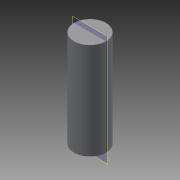
# Autodesk Inventor part: solenoid_body
Saved by Autodesk Inventor 2015 (Build 190159000, 159)
## iProperties
Created: 2015-09-23
Part Number: solenoid_body
Material: Generic
Description: insert part description/title
Document SubType Name: Modeling
Designer: francis
Density: 1 g/cm^3
Appearance: Default
Part Category: insert part category here and press enter to fill value
Author: francis
Autodesk Inventor part; units mm, degrees
ref_plane "YZ Plane" through (0, 0, 0) normal (1, 0, 0) x (0, 1, 0)
ref_plane "XY Plane" through (0, 0, 0) normal (0, 0, 1) x (1, 0, 0)
sketch "Sketch1" plane through (0, 0, 0) normal (1, 0, 0) x (0, 1, 0)
  line L0 (0, -54.8873) -> (0, 55.2482)
  line L1 (0, 55.8624) -> (24.75, 55.8624)
  line L2 (24.75, 55.8624) -> (24.75, -93.6376)
  line L3 (24.75, -93.6376) -> (7.5, -93.6376)
  line L4 (7.5, -93.6376) -> (7.5, -96.6376)
  line L5 (7.5, -96.6376) -> (10, -98.6376)
  line L6 (10, -98.6376) -> (10, -99.6376)
  line L7 (10, -99.6376) -> (0, -99.6376)
  line L8 (0, -99.6376) -> (0, 55.8624)
  point P0 (0, 0)
  dimension "d0" = 155.5
  dimension "d1" = 24.75
  dimension "d2" = 7.5
  dimension "d3" = 10
  dimension "d4" = 6
  dimension "d5" = 1
  dimension "d6" = 2
  constraints: 18 end point, 3 perpendicular, 2 vertical, 1 collinear, 1 horizontal, 1 parallel, 1 point on line
  measures "d0" distance between parallel lines of L7 L1
  measures "d1" distance of L1.start L1.end
  measures "d2" distance between parallel lines of L8 L4
  measures "d3" distance between parallel lines of L8 L6
  measures "d4" distance between parallel lines of L3 L7
  measures "d5" distance of L5.end L6.end
  measures "d6" vertical distance of L5.end L4.end
revolve "Revolution1" add sketch "Sketch1" angle 360 about axis through (0, 0, -54.8873) along (0, 0, 1)
hole "Hole1" at (0, 0, -99.6376) direction (0, 0, 1) diameter 6 depth 53.5
body "Solid1"
